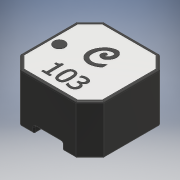
# Autodesk Inventor part: Inductor_6060
Saved by Autodesk Inventor 2018 (Build 220112000, 112)
## iProperties
Created: 2018-11-29
Part Number: Inductor_6060
Material: Copper
Document SubType Name: Modeling
Designer: Bradley
Mass: 0.48 g
Surface Area: 1.5271 cm^2
Volume: 0.112707 cm^3
Density: 4.25883 g/cm^3
Appearance: Smooth - Black
Author: Bradley
Autodesk Inventor part; units mm, degrees
ref_plane "YZ Plane" through (0, 0, 0) normal (1, 0, 0) x (0, 1, 0)
ref_plane "XZ Plane" through (0, 0, 0) normal (0, 1, 0) x (-1, 0, 0)
ref_plane "XY Plane" through (0, 0, 0) normal (0, 0, 1) x (1, 0, 0)
sketch "Sketch1" plane through (0, 0, 0) normal (0, 0, 1) x (1, 0, 0)
  line L0 (-2, -3) -> (2, -3)
  line L1 (3, -2) -> (3, 2)
  line L2 (2, 3) -> (-2, 3)
  line L3 (-3, 2) -> (-3, -2)
  line L4 (-3, -3) -> (3, 3) construction
  line L5 (3, -3) -> (-3, 3) construction
  line L6 (-2, 3) -> (-3, 2)
  line L7 (-3, -2) -> (-2, -3)
  line L8 (2, -3) -> (3, -2)
  line L9 (3, 2) -> (2, 3)
  point P0 (0, 0)
  dimension "d0" = 6
  dimension "d1" = 1
  constraints: 20 end point, 9 perpendicular, 8 point on line, 2 midpoint, 2 parallel, 1 horizontal
  measures "d0" distance of L5.end L4.end
  measures "d1" distance of L2.end L5.end
extrude "Extrusion1" add sketch "Sketch1" along normal mid plane 3.5
sketch "Sketch2" plane through (0, 0, -1.75) normal (0, 0, -1) x (-1, 0, 0)
  line L0 (3, 2) -> (2, 3) projected
  line L1 (2, 3) -> (-2, 3) projected
  line L2 (-2, 3) -> (-3, 2) projected
  line L3 (-3, 2) -> (-3, -2) projected
  line L4 (-3, -2) -> (-2, -3) projected
  line L5 (-2, -3) -> (2, -3) projected
  line L6 (2, -3) -> (3, -2) projected
  line L7 (3, -2) -> (3, 2) projected
  line L8 (2, -3) -> (-2, -3) projected
  line L9 (1, -3) -> (1, -2.3)
  line L10 (1, -2.3) -> (2.3, -2.3)
  line L11 (2.3, -2.3) -> (2.3, 2.3)
  line L12 (2.3, 2.3) -> (1, 2.3)
  line L13 (1, 2.3) -> (1, 3)
  line L14 (-2, 3) -> (2, 3) projected
  line L15 (-1, 3) -> (-1, 2.3)
  line L16 (-1, 2.3) -> (-2.3, 2.3)
  line L17 (-2.3, 2.3) -> (-2.3, -2.3)
  line L18 (-2.3, -2.3) -> (-1, -2.3)
  line L19 (-1, -3) -> (-1, -2.3)
  circle A0 centre (0, 0) radius 2.25 construction
  line L20 (1, -3) -> (-1, -3) construction
  point P0 (2.3, 0)
  point P1 (-2.3, 0)
  point P2 (0, -3)
  dimension "d11" = 2
  dimension "d12" = 0.7
  dimension "d13" = 0.7
  dimension "d14" = 4.5
  constraints: 22 end point, 12 point on line, 6 perpendicular, 4 midpoint, 2 collinear, 2 horizontal alignment, 1 centre point, 1 coincident, 1 parallel
  measures "d11" distance between parallel lines of L19 L9
  measures "d12" distance between parallel lines of L10 L5
  measures "d13" distance between parallel lines of L7 L11
  measures "d14" diameter of A0
extrude "Extrusion2" cut sketch "Sketch2" against normal blind 0.5 contours L13 L12 L11 L10 L9 L5 L19 L18 L17 L16 L15 L1
sketch "Sketch3" plane through (0, 0, -1.25) normal (0, 0, -1) x (-1, 0, 0)
  circle A0 centre (0, 0) radius 2.25 projected
extrude "Extrusion3" add sketch "Sketch3" along normal blind 0.4
fillet "Fillet1" radius 0.1 1 edges at (2.25, 0, -1.65)
sketch "Sketch4" plane through (0, 0, 1.75) normal (0, 0, 1) x (1, 0, 0)
  line L0 (-2, 3) -> (-3, 2) projected
  line L1 (-3, 2) -> (-3, -2) projected
  line L2 (-3, -2) -> (-2, -3) projected
  line L3 (-2, -3) -> (2, -3) projected
  line L4 (2, -3) -> (3, -2) projected
  line L5 (3, -2) -> (3, 2) projected
  line L6 (3, 2) -> (2, 3) projected
  line L7 (2, 3) -> (-2, 3) projected
  line L8 (-1.9172, 2.8) -> (-2.8, 1.9172)
  line L9 (-2.8, 1.9172) -> (-2.8, -1.9172)
  line L10 (-2.8, -1.9172) -> (-1.9172, -2.8)
  line L11 (-1.9172, -2.8) -> (1.9172, -2.8)
  line L12 (1.9172, -2.8) -> (2.8, -1.9172)
  line L13 (2.8, -1.9172) -> (2.8, 1.9172)
  line L14 (2.8, 1.9172) -> (1.9172, 2.8)
  line L15 (1.9172, 2.8) -> (-1.9172, 2.8)
  spline S0 degree 4 poles (-0.4296, 1.3361) (-0.247, 1.5803) (-0.0053, 1.6121) (0.3256, 1.9055) (0.7715, 1.3442) (0.6083, 0.9111) (0.3577, 0.6183) (-0.0096, 0.6513) (-0.1869, 0.8591) (-0.0066, 1.2334) (0.2137, 1.0706) (0.1689, 0.9999) (0.0758, 0.8329) (0.3431, 0.9369) (0.4135, 1.1033) (0.4648, 1.4017) (0.1427, 1.4845) (-0.2984, 1.2675) (-0.4521, 0.8147) (-0.507, 0.2278) (0.2566, -0.0734) (0.4738, 0.267) (0.692, 0.3673) (0.7727, 0.4591) knots 0 0 0 0 0 0.125046 0.175875 0.22832 0.281458 0.331424 0.378078 0.419866 0.456108 0.48813 0.516297 0.546966 0.58237 0.624695 0.65963 0.700917 0.748211 0.798236 0.861708 0.920398 1 1 1 1 1
  line L16 (0.6347, 0.3021) -> (0.9108, 0.6161) construction
  arc A0 (0.6474, 0.3673) -> (0.8477, 0.5952) centre (0.5024, 0.6968) ccw construction
  spline S1 degree 4 poles (-0.4296, 1.3361) (-0.5543, 1.1788) (-0.8408, 0.7934) (-0.7471, -0.1077) (0.1632, -0.2788) (0.6402, 0.0055) (0.7727, 0.1538) knots 0 0 0 0 0 0.459598 0.669739 1 1 1 1 1
  line L17 (0.6331, -0.0024) -> (0.9124, 0.3101) construction
  arc A1 (0.6477, 0.0518) -> (0.8602, 0.2895) centre (0.3874, 0.4983) ccw construction
  line L18 (0.7727, 0.4591) -> (0.7727, 0.1538)
  line L19 (0.2272, 1.4819) -> (-0.2269, 1.2942) construction
  arc A2 (0.1848, 1.4354) -> (-0.164, 1.2912) centre (0.2588, 0.7623) ccw construction
  circle A3 centre (-2.2, 0) radius 0.4
  line L20 (-0.5835, -2.3) -> (-1.1689, -2.3)
  line L21 (-1.1689, -2.3) -> (-1.1689, -2.1775)
  line L22 (-1.1689, -2.1775) -> (-0.9511, -2.1775)
  line L23 (-0.9511, -2.1775) -> (-0.9511, -1.3733)
  line L24 (-0.9511, -1.3733) -> (-1.1689, -1.3733)
  line L25 (-1.1689, -1.3733) -> (-1.1689, -1.2634)
  spline S2 degree 2 poles (-1.1689, -1.2634) (-1.0454, -1.2634) (-0.9287, -1.1934) (-0.9209, -1.0961) knots 0 0 0 1 2 2 2
  line L26 (-0.9209, -1.0961) -> (-0.7964, -1.0961)
  line L27 (-0.7964, -1.0961) -> (-0.7964, -2.1775)
  line L28 (-0.7964, -2.1775) -> (-0.5835, -2.1775)
  line L29 (-0.5835, -2.1775) -> (-0.5835, -2.3)
  spline S3 degree 2 poles (0.3841, -1.7) (0.3841, -2.0229) (0.1964, -2.3253) (0.001, -2.3253) knots 0 0 0 1 2 2 2
  spline S4 degree 2 poles (0.001, -2.3253) (-0.1974, -2.3253) (-0.3831, -2.017) (-0.3831, -1.701) knots 0 0 0 1 2 2 2
  spline S5 degree 2 poles (-0.3831, -1.701) (-0.3831, -1.3762) (-0.1955, -1.0757) (0.001, -1.0757) knots 0 0 0 1 2 2 2
  spline S6 degree 2 poles (0.001, -1.0757) (0.1984, -1.0757) (0.3841, -1.3869) (0.3841, -1.7) knots 0 0 0 1 2 2 2
  spline S7 degree 2 poles (0.178, -2.0656) (0.2013, -2.0063) (0.2207, -1.8235) (0.2207, -1.7) knots 0 0 0 1 2 2 2
  spline S8 degree 2 poles (0.2207, -1.7) (0.2207, -1.5765) (0.2013, -1.3947) (0.177, -1.3334) knots 0 0 0 1 2 2 2
  spline S9 degree 2 poles (0.177, -1.3334) (0.1527, -1.2721) (0.0681, -1.2089) (0.001, -1.2089) knots 0 0 0 1 2 2 2
  spline S10 degree 2 poles (0.001, -1.2089) (-0.0661, -1.2089) (-0.1527, -1.2721) (-0.178, -1.3353) knots 0 0 0 1 2 2 2
  spline S11 degree 2 poles (-0.178, -1.3353) (-0.2023, -1.3966) (-0.2198, -1.5833) (-0.2198, -1.701) knots 0 0 0 1 2 2 2
  spline S12 degree 2 poles (-0.2198, -1.701) (-0.2198, -1.8274) (-0.2042, -1.9966) (-0.1789, -2.0627) knots 0 0 0 1 2 2 2
  spline S13 degree 2 poles (-0.1789, -2.0627) (-0.1556, -2.125) (-0.069, -2.1921) (0.001, -2.1921) knots 0 0 0 1 2 2 2
  spline S14 degree 2 poles (0.001, -2.1921) (0.0671, -2.1921) (0.1536, -2.1288) (0.178, -2.0656) knots 0 0 0 1 2 2 2
  spline S15 degree 2 poles (0.8616, -1.2138) (0.8178, -1.2138) (0.7313, -1.2352) (0.6895, -1.2517) knots 0 0 0 1 2 2 2
  spline S16 degree 2 poles (0.6895, -1.2517) (0.6506, -1.2682) (0.5932, -1.3032) (0.5708, -1.3188) knots 0 0 0 1 2 2 2
  line L30 (0.5708, -1.3188) -> (0.5611, -1.3188)
  line L31 (0.5611, -1.3188) -> (0.5611, -1.1486)
  spline S17 degree 2 poles (0.5611, -1.1486) (0.6136, -1.1204) (0.7935, -1.0747) (0.8742, -1.0747) knots 0 0 0 1 2 2 2
  spline S18 degree 2 poles (0.8742, -1.0747) (0.9559, -1.0747) (1.0775, -1.1078) (1.1271, -1.1428) knots 0 0 0 1 2 2 2
  spline S19 degree 2 poles (1.1271, -1.1428) (1.1796, -1.1807) (1.234, -1.2906) (1.234, -1.3645) knots 0 0 0 1 2 2 2
  spline S20 degree 2 poles (1.234, -1.3645) (1.234, -1.4637) (1.1037, -1.6135) (1.0123, -1.6329) knots 0 0 0 1 2 2 2
  line L32 (1.0123, -1.6329) -> (1.0123, -1.6446)
  spline S21 degree 2 poles (1.0123, -1.6446) (1.0502, -1.6524) (1.1368, -1.6874) (1.1737, -1.7224) knots 0 0 0 1 2 2 2
  spline S22 degree 2 poles (1.1737, -1.7224) (1.2107, -1.7564) (1.2574, -1.8653) (1.2574, -1.9441) knots 0 0 0 1 2 2 2
  spline S23 degree 2 poles (1.2574, -1.9441) (1.2574, -2.0248) (1.2019, -2.1619) (1.1514, -2.2144) knots 0 0 0 1 2 2 2
  spline S24 degree 2 poles (1.1514, -2.2144) (1.0989, -2.2689) (0.9501, -2.3253) (0.8558, -2.3253) knots 0 0 0 1 2 2 2
  spline S25 degree 2 poles (0.8558, -2.3253) (0.7653, -2.3253) (0.5883, -2.2815) (0.528, -2.2514) knots 0 0 0 1 2 2 2
  line L33 (0.528, -2.2514) -> (0.528, -2.0812)
  line L34 (0.528, -2.0812) -> (0.5397, -2.0812)
  spline S26 degree 2 poles (0.5397, -2.0812) (0.5903, -2.1182) (0.7614, -2.1862) (0.846, -2.1862) knots 0 0 0 1 2 2 2
  spline S27 degree 2 poles (0.846, -2.1862) (0.8956, -2.1862) (0.9948, -2.1551) (1.0279, -2.1191) knots 0 0 0 1 2 2 2
  spline S28 degree 2 poles (1.0279, -2.1191) (1.06, -2.0831) (1.094, -1.9976) (1.094, -1.9324) knots 0 0 0 1 2 2 2
  spline S29 degree 2 poles (1.094, -1.9324) (1.094, -1.8673) (1.0561, -1.7827) (1.022, -1.7583) knots 0 0 0 1 2 2 2
  spline S30 degree 2 poles (1.022, -1.7583) (0.988, -1.734) (0.8956, -1.7156) (0.8412, -1.7156) knots 0 0 0 1 2 2 2
  line L35 (0.8412, -1.7156) -> (0.7731, -1.7156)
  line L36 (0.7731, -1.7156) -> (0.7731, -1.5823)
  line L37 (0.7731, -1.5823) -> (0.8266, -1.5823)
  spline S31 degree 2 poles (0.8266, -1.5823) (0.9345, -1.5823) (1.0707, -1.4793) (1.0707, -1.381) knots 0 0 0 1 2 2 2
  spline S32 degree 2 poles (1.0707, -1.381) (1.0707, -1.3353) (1.0357, -1.2702) (1.0075, -1.2507) knots 0 0 0 1 2 2 2
  spline S33 degree 2 poles (1.0075, -1.2507) (0.9773, -1.2303) (0.9034, -1.2138) (0.8616, -1.2138) knots 0 0 0 1 2 2 2
  point P0 (0, 0)
  point P1 (0, 0)
  point P2 (-0.1156, 1.5967)
  point P3 (0.1453, 1.6972)
  point P4 (0.4086, 1.6844)
  point P5 (0.6661, 1.3597)
  point P6 (0.5713, 0.9119)
  point P7 (0.2961, 0.6727)
  point P8 (0, 0.7039)
  point P9 (-0.1113, 0.9236)
  point P10 (0.0563, 1.1392)
  point P11 (0.1762, 1.0618)
  point P12 (0.159, 0.9807)
  point P13 (0.1342, 0.8941)
  point P14 (0.2502, 0.9152)
  point P15 (0.4009, 1.1072)
  point P16 (0.3862, 1.3647)
  point P17 (0.0001, 1.3881)
  point P18 (-0.4004, 0.911)
  point P19 (-0.3484, 0.2938)
  point P20 (0.1716, 0.0836)
  point P21 (0.5197, 0.2608)
  point P22 (-0.6184, 1.0437)
  point P23 (-0.7192, 0.5422)
  point P24 (-0.4891, 0.0365)
  point P25 (0.1328, -0.156)
  dimension "d0" = 6
  dimension "d1" = 1
  dimension "d20" = 0.2
  dimension "d21" = 0.8
  dimension "d22" = 2.2
  constraints: 24 end point, 6 midpoint, 4 centre point, 3 point on circle, 1 horizontal, 1 horizontal alignment, 41 other
  measures "d20" distance between parallel lines of L7 L15
  measures "d21" diameter of A3
  measures "d22" distance of point (0, 0) A3.centre
extrude "Extrusion4" cut sketch "Sketch4" against normal blind 0.02 contours L15 L14 L13 L12 L11 L10 L9 L8 | L20 L21 L22 L23 L24 L25 S2 L26 L27 L28 L29 | S3 S4 S5 S6 | S14 S13 S12 S11 S10 S9 S8 S7 | S15 S16 L30 L31 S17 S18 S19 S20 L32 S21 S22 S23 S24 S25 L33 L34 S26 S27 S28 S29 S30 L35 L36 L37 S31 S32 S33
extrude "Extrusion5" add sketch "Sketch4" against normal up to surface (0.02 mm away) contours L20 L21 L22 L23 L24 L25 S2 L26 L27 L28 L29 | S3 S4 S5 S6 | S15 S16 L30 L31 S17 S18 S19 S20 L32 S21 S22 S23 S24 S25 L33 L34 S26 S27 S28 S29 S30 L35 L36 L37 S31 S32 S33
fillet "Fillet2" radius 0.1 60 edges at (-2.5, 2.5, 1.75) (-3, 0, 1.75) (-2.5, -2.5, 1.75) (0, -3, 1.75) (2.5, -2.5, 1.75) (3, 0, 1.75) (2.5, 2.5, 1.75) (0, 3, 1.75) (1.5, 3, -1.75) (2.5, 2.5, -1.75) (3, 0, -1.75) (2.5, -2.5, -1.75) (1.5, -3, -1.75) (-1.5, -3, -1.75) (-2.5, -2.5, -1.75) (-3, 0, -1.75) (-2.5, 2.5, -1.75) (-1.5, 3, -1.75) (2, -3, 0) (-2, -3, 0) (-2, 3, 0) (2, 3, 0) (3, 2, 0) (3, -2, 0) (-3, -2, 0) (-3, 2, 0) (1, -2.65, -1.25) (1, -2.3, -1.5) (1.65, -2.3, -1.25) (2.3, -2.3, -1.5) (2.3, 0, -1.25) (2.3, 2.3, -1.5) (1.65, 2.3, -1.25) (1, 2.3, -1.5) (1, 2.65, -1.25) (-1, -2.65, -1.25) (-1.65, -2.3, -1.25) (-2.3, 0, -1.25) (-1.65, 2.3, -1.25) (-1, 2.65, -1.25) (-1, -2.3, -1.5) (-2.3, -2.3, -1.5) (-2.3, 2.3, -1.5) (-1, 2.3, -1.5) (-1, -3, -1.5) (0, -3, -1.25) (1, -3, -1.5) (1, -2.65, -1.75) (-1, -2.65, -1.75) (-1.65, -2.3, -1.75) (-2.3, 0, -1.75) (-1.65, 2.3, -1.75) (-1, 2.65, -1.75) (-1, 3, -1.5) (0, 3, -1.25) (1, 2.65, -1.75) (1, 3, -1.5) (1.65, 2.3, -1.75) (2.3, 0, -1.75) (1.65, -2.3, -1.75)
equation "\"d13\" = d12"
body "Solid1"
